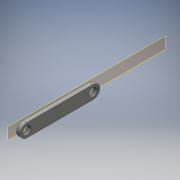
# Autodesk Inventor part: ArmSpan_015
Saved by Autodesk Inventor 2016 (Build 200138000, 138)
## iProperties
Created: 2016-11-02
Part Number: ArmSpan_015
Material: Generic
Document SubType Name: Modeling
Designer: mattc
Density: 1 g/cm^3
Appearance: Smooth - Medium Gray
Author: mattc
Autodesk Inventor part; units mm, degrees
ref_plane "YZ Plane" through (0, 0, 0) normal (1, 0, 0) x (0, 1, 0)
ref_plane "XZ Plane" through (0, 0, 0) normal (0, 1, 0) x (-1, 0, 0)
ref_plane "XY Plane" through (0, 0, 0) normal (0, 0, 1) x (1, 0, 0)
sketch "Sketch1" plane through (0, 0, 0) normal (1, 0, 0) x (0, 1, 0)
  circle A0 centre (0, 0) radius 3.1
  arc A1 (0, 5) -> (0, -5) centre (0, 0) ccw
  line L0 (0, 5) -> (50, 5)
  line L1 (50, -5) -> (0, -5)
  arc A2 (50, -5) -> (50, 5) centre (50, 0) ccw
  circle A3 centre (50, 0) radius 3.1
  dimension "d0" = 6.2
  dimension "d1" = 10
  dimension "d3" = 50
  dimension "d5" = 6.2
  dimension "d26" = 5
  constraints: 4 centre point, 4 end point, 4 point on circle, 3 coincident, 3 tangent, 1 horizontal, 1 parallel
  measures "d0" diameter of A0
  measures "d1" diameter of A1
  measures "d3" distance of L0.start L0.end
  measures "d5" diameter of A3
  measures "d26" radius of A2
extrude "Extrusion1" add sketch "Sketch1" along normal blind 3
ref_plane "Work Plane1" through (-2, 0, 0) normal (1, 0, 0) x (0, 0, -1)
equation "\"d5\" = d0"
equation "\"d26\" = 0.5 * d1"
body "Solid1"
